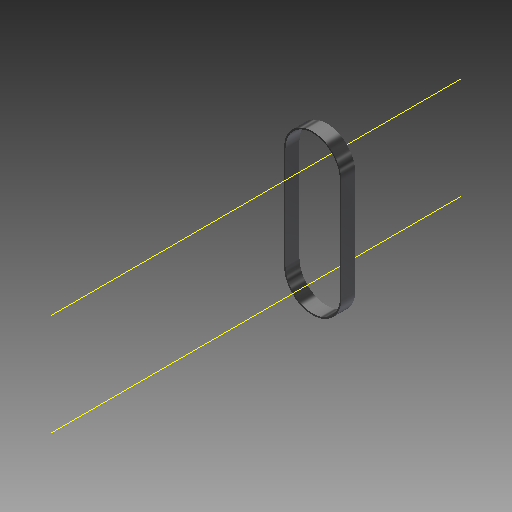
# Autodesk Inventor part: Synchronous Belt
Saved by Autodesk Inventor 2019.4 (Build 234330000, 330)
## iProperties
Created: 2019-11-29
Part Number: Synchronous Belt
Material: Aluminum 6061
Document SubType Name: Modeling
Designer: admin
Mass: 2.418 g
Surface Area: 57.2 cm^2
Volume: 2.6 cm^3
Density: 2.7 g/cm^3
Appearance: Aluminum - Flat
CustomPartVersion: 0
Author: admin
Autodesk Inventor part; units mm, degrees
ref_plane "YZ Plane" through (0, 0, 0) normal (1, 0, 0) x (0, 1, 0)
ref_plane "XZ Plane" through (0, 0, 0) normal (0, 1, 0) x (-1, 0, 0)
ref_plane "XY Plane" through (0, 0, 0) normal (0, 0, 1) x (1, 0, 0)
sketch "Sketch Path" plane through (0, 0, 0) normal (0, 0, 1) x (1, 0, 0)
  arc A0 (19.8944, 19.6444) -> (-19.8944, 19.6444) centre (0, 19.6444) ccw
  arc A1 (-19.8944, -52.8556) -> (19.8944, -52.8556) centre (0, -52.8556) ccw
  line L0 (-19.8944, -52.8556) -> (-19.8944, 19.6444)
  line L1 (19.8944, 19.6444) -> (19.8944, -52.8556)
  constraints: 4 end point, 4 point on circle, 2 centre point
ref_plane "Cross Section Plane" through (-19.8944, 19.6444, 0) normal (0, -1, 0) x (0, 0, 1)
ref_plane "Work Plane2" through (0, 19.6444, 0) normal (-1, 0, 0) x (0, 0, 1)
ref_plane "Work Plane3" through (0, -52.8556, 0) normal (0.0627905, 0.9980267, 0) x (0, 0, 1)
sketch "Cross Section" plane through (-19.8944, 19.6444, 0) normal (0, -1, 0) x (0, 0, 1)
  line L0 (-5, 0.5) -> (5, 0.5)
  line L1 (5, 0.5) -> (5, -0.5)
  line L2 (5, -0.5) -> (-5, -0.5)
  line L3 (-5, -0.5) -> (-5, 0.5)
  line L4 (-5, 0) -> (5, 0) construction
  point P0 (0, 0)
  point P1 (0, 0)
  dimension "d0" = 10
  dimension "d4" = 0.5
  dimension "d5" = 0.5
  constraints: 10 end point, 3 midpoint, 2 parallel, 1 coincident, 1 horizontal, 1 perpendicular, 1 other
  measures "d0" distance between parallel lines of L1 L3
  measures "d4" distance between parallel lines of L2 L4
  measures "d5" distance between parallel lines of L4 L0
sweep "Belt" add profiles "Cross Section" path "Sketch Path" path curves L1 A1 L0 A0
equation "\"d0\" = da_B"
equation "\"d4\" = da_a"
equation "\"d5\" = da_a2"
equation "\"da_B\" = 10"
equation "\"da_pb\" = 5"
equation "\"da_a\" = 0.5"
equation "\"da_S\" = 2.65"
equation "\"da_Beta\" = 20deg"
equation "\"da_Ht\" = 1.2"
equation "\"da_H\" = 2.2"
equation "\"da_a2\" = 0.5"
body "Solid1"
